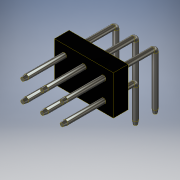
# Autodesk Inventor part: conn_2x3_2mm_RA
Saved by Autodesk Inventor 2016 (Build 200138000, 138)
## iProperties
Created: 2016-09-12
Part Number: conn_2x3_2mm_RA
Material: Generic
Document SubType Name: Modeling
Designer: jfixelle
Density: 1 g/cm^3
Appearance: Silver
Author: jfixelle
Autodesk Inventor part; units mm, degrees
ref_plane "YZ Plane" through (0, 0, 0) normal (1, 0, 0) x (0, 1, 0)
ref_plane "XZ Plane" through (0, 0, 0) normal (0, 1, 0) x (-1, 0, 0)
ref_plane "XY Plane" through (0, 0, 0) normal (0, 0, 1) x (1, 0, 0)
sketch "Sketch1" plane through (0, 0, 0) normal (0, 0, 1) x (1, 0, 0)
  line L0 (-3, 4) -> (3, 4)
  line L1 (3, 4) -> (3, 0)
  line L2 (3, 0) -> (-3, 0)
  line L3 (-3, 0) -> (-3, 4)
  point P0 (0, 0)
  dimension "d0" = 6
  dimension "d1" = 3
  dimension "d2" = 4
  dimension "d3" = 0
  constraints: 8 end point, 2 parallel, 1 horizontal, 1 perpendicular
  measures "d0" distance of L0.start L0.end
  measures "d1" distance from line of L1 point (0, 0)
  measures "d2" distance of L0.end L1.end
  measures "d3" distance from line of L2 point (0, 0)
extrude "Extrusion1" add sketch "Sketch1" along normal blind 1.5
sketch "Sketch2" plane through (0, 0, 0) normal (1, 0, 0) x (0, 1, 0)
  line L0 (3.05, 5.75) -> (3.05, -3.45)
  line L1 (2.75, -3.75) -> (-2.65, -3.75)
  line L2 (1.05, 5.75) -> (1.05, -1.45)
  line L3 (0.75, -1.75) -> (-2.65, -1.75)
  line L4 (0, 1.5) -> (4, 1.5) projected
  line L5 (0, 0) -> (0, 1.5) projected
  arc A0 (0.75, -1.75) -> (1.05, -1.45) centre (0.75, -1.45) ccw
  arc A1 (2.75, -3.75) -> (3.05, -3.45) centre (2.75, -3.45) ccw
  dimension "d6" = 4.25
  dimension "d7" = 4.25
  dimension "d8" = 2.65
  dimension "d9" = 2.65
  dimension "d10" = 2
  dimension "d11" = 3.25
  dimension "d12" = 2
  dimension "d13" = 1.05
  dimension "d14" = 0.3
  constraints: 8 end point, 4 point on circle, 4 tangent, 2 centre point, 2 perpendicular, 2 vertical, 1 equal radius
  measures "d6" distance from line of L4 L0.start
  measures "d7" distance from line of L4 L2.start
  measures "d8" distance from line of L3.end L5
  measures "d9" distance from line of L5 L1.end
  measures "d10" distance between parallel lines of L1 L3
  measures "d11" distance between parallel lines of L4 L3
  measures "d12" distance between parallel lines of L2 L0
  measures "d13" distance between parallel lines of L5 L2
  measures "d14" radius of A0
sketch "Sketch3" plane through (0, 0, 0) normal (0, 1, 0) x (-1, 0, 0)
  circle A0 centre (0, -3.75) radius 0.25
  line L0 (0, 0) -> (0, -0.006)
  line L1 (3, 0) -> (-3, 0) projected
  circle A1 centre (0, -1.75) radius 0.25
  line L2 (-3, 1.5) -> (3, 1.5) projected
  dimension "d16" = 3.25
  dimension "d17" = 2
  dimension "d18" = 0.5
  dimension "d19" = 0.5
  constraints: 2 centre point, 2 end point, 1 vertical
  measures "d16" distance from line of L2 A1.centre
  measures "d17" distance of A0.centre A1.centre
  measures "d18" diameter of A1
  measures "d19" diameter of A0
sketch "Sketch4" plane through (0, 0, 0) normal (1, 0, 0) x (0, 1, 0)
  line L0 (3.05, 5.75) -> (3.05, -3.45)
  line L1 (2.75, -3.75) -> (-2.65, -3.75)
  line L2 (0, 0) -> (0, 1.5) projected
  line L3 (0, 1.5) -> (4, 1.5) projected
  arc A0 (2.75, -3.75) -> (3.05, -3.45) centre (2.75, -3.45) ccw
  dimension "d20" = 3.05
  dimension "d21" = 4.25
  dimension "d22" = 5.25
  dimension "d23" = 2.65
  dimension "d24" = 0.3
  constraints: 4 end point, 2 point on circle, 2 tangent, 1 centre point, 1 perpendicular, 1 vertical
  measures "d20" distance between parallel lines of L2 L0
  measures "d21" distance from line of L3 L0.start
  measures "d22" distance between parallel lines of L3 L1
  measures "d23" distance from line of L2 L1.end
  measures "d24" radius of A0
sketch "Sketch5" plane through (0, 0, 0) normal (0, 1, 0) x (-1, 0, 0)
  circle A0 centre (0, -3.75) radius 0.25
  line L0 (-3, 1.5) -> (3, 1.5) projected
  point P0 (0, 0)
  dimension "d25" = 5.25
  dimension "d26" = 0.5
  constraints: 1 centre point
  measures "d25" distance from line of L0 A0.centre
  measures "d26" diameter of A0
sweep "Sweep1" add profiles "Sketch3" path "Sketch2" path curves L2 A0 L3 contours A1
sweep "Sweep2" add profiles "Sketch5" path "Sketch4" path curves L1 A0 L0
chamfer "Chamfer1" distance 0.4 angle 10 1 edges at (0.25, 3.05, 5.75) measured on face at (-0.2492, 3.0299, 4.3333)
chamfer "Chamfer2" distance 0.4 angle 10 1 edges at (0.25, 1.05, 5.75) measured on face at (-0.2492, 1.0299, 4.3333)
chamfer "Chamfer3" distance 0.4 angle 10 1 edges at (0.25, -2.65, -3.75) measured on face at (-0.2468, 0.95, -3.7901)
chamfer "Chamfer4" distance 0.4 angle 10 1 edges at (0.25, -2.65, -1.75) measured on face at (-0.2468, -0.3833, -1.7901)
pattern_linear "Rectangular Pattern1" count 3 spacing 2 along (-1, 0, 0) of "Sweep1", "Sweep2", "Chamfer1", "Chamfer2", "Chamfer3", "Chamfer4" first direction both ways yes
body "Solid1"
